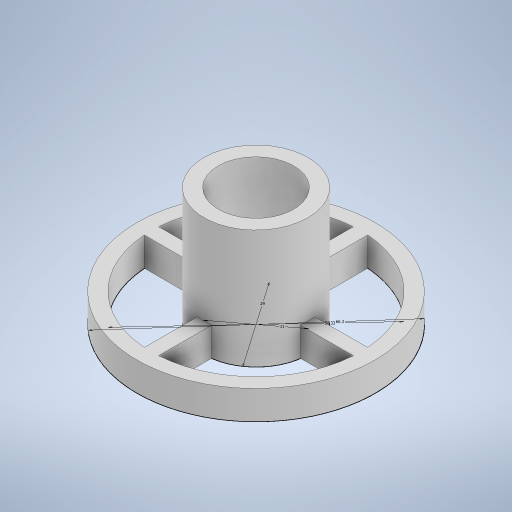
# Autodesk Inventor part: Calibrator
Saved by Autodesk Inventor 2023.2 (Build 272271030, 271C)
## iProperties
Created: 2023-05-25
Part Number: Calibrator
Material: Generic
Document SubType Name: Modeling
Designer: Lukas
Density: 1 g/cm^3
Appearance: Default
Author: Lukas
Autodesk Inventor part; units mm, degrees
ref_plane "YZ Plane" through (0, 0, 0) normal (1, 0, 0) x (0, 1, 0)
ref_plane "XZ Plane" through (0, 0, 0) normal (0, 1, 0) x (-1, 0, 0)
ref_plane "XY Plane" through (0, 0, 0) normal (0, 0, 1) x (1, 0, 0)
sketch "Sketch1" plane through (0, 0, 0) normal (0, 1, 0) x (-1, 0, 0)
  circle A0 centre (0, 0) radius 33.15
  circle A1 centre (0, 0) radius 29.165
  circle A2 centre (0, 0) radius 10.5
  circle A3 centre (0, 0) radius 14.5
  dimension "d0" = 66.3
  dimension "d1" = 58.33
  dimension "d2" = 21
  dimension "d3" = 29
  constraints: 4 centre point, 4 coincident
  measures "d0" diameter of A0
  measures "d1" diameter of A1
  measures "d2" diameter of A2
  measures "d3" diameter of A3
sketch "Sketch2" plane through (0, 0, 0) normal (0, 1, 0) x (-1, 0, 0)
  line L0 (2, 33) -> (-2, 33)
  line L1 (-2, 33) -> (-2, 12)
  line L2 (-2, 12) -> (2, 12)
  line L3 (2, 12) -> (2, 33)
  line L4 (33, 2) -> (12, 2)
  line L5 (12, 2) -> (12, -2)
  line L6 (12, -2) -> (33, -2)
  line L7 (33, -2) -> (33, 2)
  line L8 (2, -12) -> (-2, -12)
  line L9 (-2, -12) -> (-2, -33)
  line L10 (-2, -33) -> (2, -33)
  line L11 (2, -33) -> (2, -12)
  line L12 (-12, 2) -> (-33, 2)
  line L13 (-33, 2) -> (-33, -2)
  line L14 (-33, -2) -> (-12, -2)
  line L15 (-12, -2) -> (-12, 2)
  point P0 (0, 0)
  point P1 (12, 0)
  point P2 (0, -12)
  point P3 (-33, 0)
  dimension "d4" = 4
  dimension "d5" = 4
  dimension "d6" = 12
  dimension "d7" = 12
  dimension "d8" = 12
  dimension "d9" = 12
  dimension "d10" = 21
  dimension "d11" = 21
  dimension "d12" = 21
  dimension "d13" = 21
  dimension "d14" = 2
  dimension "d15" = 2
  constraints: 32 end point, 8 parallel, 4 horizontal, 4 perpendicular, 4 point on line, 3 midpoint
  measures "d4" distance between parallel lines of L1 L3
  measures "d5" distance between parallel lines of L4 L6
  measures "d6" distance of point (0, 0) point (12, 0)
  measures "d7" distance from line of L15 point (0, 0)
  measures "d8" distance of point (0, -12) point (0, 0)
  measures "d9" distance from line of L2 point (0, 0)
  measures "d10" distance between parallel lines of L0 L2
  measures "d11" distance between parallel lines of L10 L8
  measures "d12" distance between parallel lines of L7 L5
  measures "d13" distance from line of point (-33, 0) L15
  measures "d14" distance from line of point (0, 0) L12
  measures "d15" distance from line of point (0, 0) L11
extrude "Extrusion1" add sketch "Sketch1" along normal blind 8
extrude "Extrusion2" add sketch "Sketch2" along normal blind 8
extrude "Extrusion3" add sketch "Sketch1" along normal blind 33 contours A3
equation "\"d11\" = d10"
equation "\"d12\" = d10"
equation "\"d13\" = d10"
body "Solid1"
